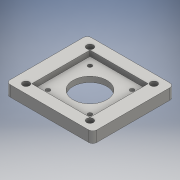
# Autodesk Inventor part: motor support
Saved by Autodesk Inventor 2016 SP1 (Build 200210100, 210)
## iProperties
Created: 2016-04-14
Part Number: motor support
Material: Generic
Document SubType Name: Modeling
Designer: ubik
Density: 1 g/cm^3
Appearance: Default
Author: ubik
Autodesk Inventor part; units mm, degrees
ref_plane "YZ Plane" through (0, 0, 0) normal (1, 0, 0) x (0, 1, 0)
ref_plane "XZ Plane" through (0, 0, 0) normal (0, 1, 0) x (-1, 0, 0)
ref_plane "XY Plane" through (0, 0, 0) normal (0, 0, 1) x (1, 0, 0)
sketch "Sketch1" plane through (0, 0, 0) normal (0, 0, 1) x (1, 0, 0)
  circle A0 centre (0, 0) radius 12.5
  circle A1 centre (-15.4996, 15.5) radius 1.5
  circle A2 centre (-15.5, -15.4996) radius 1.5
  circle A3 centre (15.4996, -15.5) radius 1.5
  circle A4 centre (15.5, 15.4996) radius 1.5
  circle A5 centre (-23.5679, 23.5679) radius 2.5
  circle A6 centre (-23.5679, -23.5679) radius 2.5
  circle A7 centre (23.5679, -23.5679) radius 2.5
  circle A8 centre (23.5679, 23.5679) radius 2.5
  line L0 (0, 0) -> (-27.3582, 27.3582) construction
  line L1 (-32, 30) -> (32, 30)
  line L2 (32, 30) -> (32, -30)
  line L3 (32, -30) -> (-32, -30)
  line L4 (-32, -30) -> (-32, 30)
  dimension "d0" = 3
  dimension "d1" = 21.92
  dimension "d4" = 360
  dimension "d6" = 15.5
  dimension "d7" = 25
  dimension "d8" = 5
  dimension "d9" = 33.33
  dimension "d12" = 360
  dimension "d14" = 0
  dimension "d15" = 64
  dimension "d16" = 60
  dimension "d17" = 30
  dimension "d18" = 32
  constraints: 10 end point, 9 centre point, 2 parallel, 1 coincident, 1 horizontal, 1 perpendicular, 18 other
  measures "d0" diameter of A1
  measures "d1" distance of point (0, 0) A1.centre
  measures "d6" vertical distance of point (0, 0) A1.centre
  measures "d7" diameter of A0
  measures "d8" diameter of A5
  measures "d9" distance of point (0, 0) A5.centre
  measures "d14" distance from line of L0 A5.centre
  measures "d15" distance of L1.start L1.end
  measures "d16" distance of L3.end L1.start
  measures "d17" distance from line of point (0, 0) L1
  measures "d18" distance from line of point (0, 0) L4
extrude "Extrusion1" add sketch "Sketch1" along normal blind 8
sketch "Sketch2" plane through (0, 0, 8) normal (0, 0, 1) x (1, 0, 0)
  line L0 (-21.5, 21.5) -> (21.5, 21.5)
  line L1 (21.5, 21.5) -> (21.5, -21.5)
  line L2 (21.5, -21.5) -> (-21.5, -21.5)
  line L3 (-21.5, -21.5) -> (-21.5, 21.5)
  point P0 (0, 0)
  dimension "d21" = 43
  dimension "d22" = 43
  dimension "d23" = 21.5
  dimension "d24" = 21.5
  constraints: 8 end point, 2 parallel, 1 horizontal, 1 perpendicular
  measures "d21" distance of L0.start L0.end
  measures "d22" distance of L2.end L0.start
  measures "d23" distance from line of point (0, 0) L0
  measures "d24" distance from line of point (0, 0) L3
extrude "Extrusion2" cut sketch "Sketch2" against normal blind 4
fillet "Fillet1" radius 3 4 edges at (32, 30, 4) (-32, 30, 4) (-32, -30, 4) (32, -30, 4)
equation "\"d17\" = 0.5 * d16"
equation "\"d18\" = 0.5 * d15"
equation "\"d21\" = d22"
equation "\"d23\" = 0.5 * d22"
equation "\"d24\" = 0.5 * d21"
body "Solid1"
